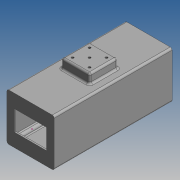
# Autodesk Inventor part: P033_Boitier_v3
Saved by Autodesk Inventor 2021.3 (Build 253353000, 353)
## iProperties
Created: 2021-11-26
Part Number: P033_Boitier_v3
Material: Générique
Document SubType Name: Modeling
Designer: gabri
Density: 1 g/cm^3
Appearance: Par défaut
Author: gabri
Autodesk Inventor part; units mm, degrees
ref_plane "YZ Plane" through (0, 0, 0) normal (1, 0, 0) x (0, 1, 0)
ref_plane "XZ Plane" through (0, 0, 0) normal (0, 1, 0) x (-1, 0, 0)
ref_plane "XY Plane" through (0, 0, 0) normal (0, 0, 1) x (1, 0, 0)
sketch "Sketch3" plane through (0, 0, 0) normal (0, 1, 0) x (-1, 0, 0)
  line L0 (-50, -50) -> (50, -50)
  line L1 (50, -50) -> (50, 50)
  line L2 (50, 50) -> (-50, 50)
  line L3 (-50, 50) -> (-50, -50)
  line L4 (-50, -50) -> (50, 50) construction
  line L5 (50, -50) -> (-50, 50) construction
  point P0 (0, 0)
  dimension "d0" = 100
  dimension "d1" = 100
  constraints: 12 end point, 2 midpoint, 2 parallel, 1 horizontal, 1 perpendicular
  measures "d0" distance between parallel lines of L3 L1
  measures "d1" distance between parallel lines of L0 L2
extrude "Extrusion1" add sketch "Sketch3" along normal blind 250
sketch "Sketch4" plane through (0, 0, 0) normal (0, -1, 0) x (1, 0, 0)
  line L0 (34, -21.5) -> (-34, -21.5)
  line L1 (-34, -21.5) -> (-34, 21.5)
  line L2 (-34, 21.5) -> (34, 21.5)
  line L3 (34, 21.5) -> (34, -21.5)
  line L4 (34, -21.5) -> (-34, 21.5) construction
  line L5 (-34, -21.5) -> (34, 21.5) construction
  point P0 (0, 0)
  dimension "d4" = 68
  dimension "d5" = 43
  constraints: 12 end point, 2 midpoint, 2 parallel, 1 horizontal, 1 perpendicular
  measures "d4" distance of L1.end L2.end
  measures "d5" distance of L0.end L1.end
extrude "Extrusion2" cut sketch "Sketch4" against normal blind 2
shell "Shell1" thickness 3 removed faces 2 at (16.6667, 250, -16.6667) at (-11.3333, 2, -7.1667)
sketch "Sketch10" plane through (0, 250, 0) normal (0, 1, 0) x (1, 0, 0)
  line L0 (-47, 47) -> (-47, -47) construction
  line L1 (-47, -47) -> (47, -47) construction
  line L2 (47, -47) -> (47, 47) construction
  line L3 (47, 47) -> (-47, 47) construction
  line L4 (-50, -50) -> (50, -50) construction
  line L5 (50, -50) -> (50, 50) construction
  line L6 (50, 50) -> (-50, 50) construction
  line L7 (-50, 50) -> (-50, -50) construction
  circle A0 centre (45, -45) radius 5
  circle A1 centre (-45, -45) radius 5
  circle A2 centre (-45, 45) radius 5
  circle A3 centre (45, 45) radius 5
  point P0 (0, 0)
  dimension "d26" = 10
  dimension "d27" = 5
  dimension "d28" = 5
  dimension "d29" = 10
  dimension "d30" = 5
  dimension "d31" = 5
  dimension "d32" = 5
  dimension "d33" = 10
  dimension "d34" = 5
  dimension "d37" = 10
  dimension "d38" = 5
  dimension "d39" = 5
  constraints: 4 centre point
  measures "d26" diameter of A0
  measures "d27" distance from line of L4 A0.centre
  measures "d28" distance from line of A0.centre L5
  measures "d29" diameter of A1
  measures "d30" distance from line of L4 A1.centre
  measures "d31" distance from line of L7 A1.centre
  measures "d32" distance from line of L7 A2.centre
  measures "d33" diameter of A2
  measures "d34" distance from line of L6 A2.centre
  measures "d37" diameter of A3
  measures "d38" distance from line of L5 A3.centre
  measures "d39" distance from line of L6 A3.centre
extrude "Extrusion5" add sketch "Sketch10" against normal up to surface (247 mm away)
sketch "Sketch11" plane through (0, 250, 0) normal (0, 1, 0) x (1, 0, 0)
  line L0 (-40.4174, 47) -> (40.4174, 47) construction
  arc A0 (40.4174, 47) -> (47, 40.4174) centre (45, 45) ccw construction
  line L1 (47, 40.4174) -> (47, -40.4174) construction
  arc A1 (47, -40.4174) -> (40.4174, -47) centre (45, -45) ccw construction
  line L2 (40.4174, -47) -> (-40.4174, -47) construction
  arc A2 (-40.4174, -47) -> (-47, -40.4174) centre (-45, -45) ccw construction
  line L3 (-47, -40.4174) -> (-47, 40.4174) construction
  arc A3 (-47, 40.4174) -> (-40.4174, 47) centre (-45, 45) ccw construction
  line L4 (50, 50) -> (-50, 50) construction
  line L5 (-50, 50) -> (-50, -50) construction
  line L6 (-50, -50) -> (50, -50) construction
  line L7 (50, -50) -> (50, 50) construction
  arc A4 (47, -40.4174) -> (40.4174, -47) centre (45, -45) ccw
  arc A5 (-40.4174, -47) -> (-47, -40.4174) centre (-45, -45) ccw
  arc A6 (-47, 40.4174) -> (-40.4174, 47) centre (-45, 45) ccw
  arc A7 (40.4174, 47) -> (47, 40.4174) centre (45, 45) ccw
  line L8 (40.4174, 47) -> (-40.4174, 47)
  line L9 (47, -40.4174) -> (47, 40.4174)
  line L10 (40.4174, -47) -> (-40.4174, -47)
  line L11 (-47, -40.4174) -> (-47, 40.4174)
  arc A8 (48, -42.3542) -> (42.3542, -48) centre (45, -45) ccw
  line L12 (42.3542, -48) -> (-42.3542, -48)
  arc A9 (-42.3542, -48) -> (-48, -42.3542) centre (-45, -45) ccw
  line L13 (-48, -42.3542) -> (-48, 42.3542)
  arc A10 (-48, 42.3542) -> (-42.3542, 48) centre (-45, 45) ccw
  line L14 (42.3542, 48) -> (-42.3542, 48)
  arc A11 (42.3542, 48) -> (48, 42.3542) centre (45, 45) ccw
  line L15 (48, -42.3542) -> (48, 42.3542)
  point P0 (0, 0)
  dimension "d45" = 1
  dimension "d46" = 4
  dimension "d47" = 1
  dimension "d48" = 4
  dimension "d49" = 1
  dimension "d50" = 4
  dimension "d51" = 1
  dimension "d54" = 4
  constraints: 17 point on circle, 16 end point, 8 centre point, 6 parallel, 4 coincident, 4 concentric, 2 collinear
  measures "d45" distance between parallel lines of L12 L10
  measures "d46" radius of A9
  measures "d47" distance between parallel lines of L13 L3
  measures "d48" radius of A10
  measures "d49" distance between parallel lines of L14 L0
  measures "d50" radius of A11
  measures "d51" distance between parallel lines of L1 L15
  measures "d54" radius of A8
extrude "Extrusion6" add sketch "Sketch11" along normal blind 2
fillet "Fillet1" radius 2 16 edges at (40.4174, 251, 47) (40.4174, 126.5, 47) (47, 251, 40.4174) (47, 126.5, 40.4174) (-40.4174, 251, 47) (-40.4174, 126.5, 47) (-47, 251, 40.4174) (-47, 126.5, 40.4174) (-47, 251, -40.4174) (-47, 126.5, -40.4174) (-40.4174, 251, -47) (-40.4174, 126.5, -47) (40.4174, 251, -47) (40.4174, 126.5, -47) (47, 251, -40.4174) (47, 126.5, -40.4174)
fillet "Fillet2" radius 2 8 edges at (42.3542, 251, -48) (48, 251, -42.3542) (48, 251, 42.3542) (42.3542, 251, 48) (-42.3542, 251, 48) (-48, 251, 42.3542) (-42.3542, 251, -48) (-48, 251, -42.3542)
fillet "Fillet3" radius 0.5 32 edges at (41.4645, 252, 41.4645) (46.4142, 252, 39.4142) (47, 252, 0) (46.4142, 252, -39.4142) (41.4645, 252, -41.4645) (39.4142, 252, -46.4142) (0, 252, -47) (-39.4142, 252, -46.4142) (-41.4645, 252, -41.4645) (-46.4142, 252, -39.4142) (-47, 252, 0) (-46.4142, 252, 39.4142) (-41.4645, 252, 41.4645) (-39.4142, 252, 46.4142) (0, 252, 47) (39.4142, 252, 46.4142) (-40.6114, 252, -47.291) (-42.1716, 252, -42.1716) (-47.291, 252, -40.6114) (-48, 252, 0) (-47.291, 252, 40.6114) (-42.1716, 252, 42.1716) (-40.6114, 252, 47.291) (0, 252, 48) (40.6114, 252, 47.291) (42.1716, 252, 42.1716) (47.291, 252, 40.6114) (48, 252, 0) (47.291, 252, -40.6114) (42.1716, 252, -42.1716) (40.6114, 252, -47.291) (0, 252, -48)
sketch "Sketch12" plane through (0, 250, 0) normal (0, 1, 0) x (1, 0, 0)
  line L0 (-39.0839, 48) -> (39.0839, 48) construction
  arc A0 (41.0559, 45.6667) -> (39.0839, 48) centre (39.0839, 46) ccw construction
  arc A1 (41.0559, 45.6667) -> (45.6667, 41.0559) centre (45, 45) ccw construction
  arc A2 (48, 39.0839) -> (45.6667, 41.0559) centre (46, 39.0839) ccw construction
  line L1 (48, 39.0839) -> (48, -39.0839) construction
  arc A3 (45.6667, -41.0559) -> (48, -39.0839) centre (46, -39.0839) ccw construction
  arc A4 (45.6667, -41.0559) -> (41.0559, -45.6667) centre (45, -45) ccw construction
  arc A5 (39.0839, -48) -> (41.0559, -45.6667) centre (39.0839, -46) ccw construction
  line L2 (39.0839, -48) -> (-39.0839, -48) construction
  arc A6 (-41.0559, -45.6667) -> (-39.0839, -48) centre (-39.0839, -46) ccw construction
  arc A7 (-41.0559, -45.6667) -> (-45.6667, -41.0559) centre (-45, -45) ccw construction
  arc A8 (-48, -39.0839) -> (-45.6667, -41.0559) centre (-46, -39.0839) ccw construction
  line L3 (-48, -39.0839) -> (-48, 39.0839) construction
  arc A9 (-45.6667, 41.0559) -> (-48, 39.0839) centre (-46, 39.0839) ccw construction
  arc A10 (-45.6667, 41.0559) -> (-41.0559, 45.6667) centre (-45, 45) ccw construction
  arc A11 (-39.0839, 48) -> (-41.0559, 45.6667) centre (-39.0839, 46) ccw construction
  line L4 (50, 50) -> (-50, 50) construction
  line L5 (-50, 50) -> (-50, -50) construction
  line L6 (-50, -50) -> (50, -50) construction
  line L7 (50, -50) -> (50, 50) construction
  point P0 (0, 0)
  constraints: 4 coincident
hole "Hole1" at (45, 250, 45) at (-45, 250, 45) at (-45, 250, -45) at (45, 250, -45) direction (0, -1, 0) diameter 4.134 depth 14.2 tip angle 118 thread size "M5x0.8" class "6H" standard "ISO Metric profile"
fillet "Fillet4" radius 4 4 edges at (-50, 125, 50) (50, 125, 50) (50, 125, -50) (-50, 125, -50)
sketch "Sketch15" plane through (-46, 0, 50) normal (0, 0, 1) x (1, 0, 0)
  line L0 (92, 250) -> (92, 0) construction
  line L1 (0, 250) -> (92, 250) construction
  line L2 (0, 0) -> (0, 250) construction
  line L3 (0, 0) -> (92, 0) construction
  line L4 (76, 95) -> (16, 95)
  line L5 (16, 95) -> (16, 155)
  line L6 (16, 155) -> (76, 155)
  line L7 (76, 155) -> (76, 95)
  line L8 (76, 95) -> (16, 155) construction
  line L9 (16, 95) -> (76, 155) construction
  line L10 (46, 302.4) -> (46, -50.4) construction
  point P0 (46, 0)
  point P1 (46, 125)
  point P2 (46, 125)
  dimension "d67" = 60
  dimension "d68" = 60
  dimension "d69" = 250
  dimension "d70" = 125
  constraints: 12 end point, 3 midpoint, 2 parallel, 1 horizontal, 1 perpendicular, 1 point on line
  measures "d67" distance between parallel lines of L7 L5
  measures "d68" distance between parallel lines of L4 L6
  measures "d69" distance between parallel lines of L3 L1
  measures "d70" distance from line of point (46, 125) L1
extrude "Extrusion7" add sketch "Sketch15" along normal blind 20
fillet "Fillet5" radius 4 12 edges at (30, 95, 60) (30, 155, 60) (-30, 155, 60) (-30, 95, 60) (-30, 125, 50) (0, 95, 50) (30, 125, 50) (0, 155, 50) (30, 125, 70) (0, 155, 70) (-30, 125, 70) (0, 95, 70)
sketch "Sketch17" plane through (-38, 3, -47) normal (0, 1, 0) x (1, 0, 0)
  point P0 (38, -47)
sketch "Sketch18" plane through (-38, 3, -47) normal (0, 1, 0) x (1, 0, 0)
  line L0 (1, -22.5) -> (1, -71.5) construction
  line L1 (75, -22.5) -> (1, -22.5) construction
  line L2 (75, -71.5) -> (75, -22.5) construction
  line L3 (1, -71.5) -> (75, -71.5) construction
  arc A0 (85, -9) -> (83, -7) centre (83, -9) ccw construction
  arc A1 (78, -2) -> (83, -7) centre (83, -2) ccw construction
  arc A2 (78, -2) -> (76, 0) centre (76, -2) ccw construction
  line L4 (76, 0) -> (0, 0) construction
  arc A3 (0, 0) -> (-2, -2) centre (0, -2) ccw construction
  arc A4 (-7, -7) -> (-2, -2) centre (-7, -2) ccw construction
  arc A5 (-7, -7) -> (-9, -9) centre (-7, -9) ccw construction
  line L5 (-9, -9) -> (-9, -85) construction
  arc A6 (-9, -85) -> (-7, -87) centre (-7, -85) ccw construction
  arc A7 (-2, -92) -> (-7, -87) centre (-7, -92) ccw construction
  arc A8 (-2, -92) -> (0, -94) centre (0, -92) ccw construction
  line L6 (0, -94) -> (76, -94) construction
  arc A9 (76, -94) -> (78, -92) centre (76, -92) ccw construction
  arc A10 (83, -87) -> (78, -92) centre (83, -92) ccw construction
  arc A11 (83, -87) -> (85, -85) centre (83, -85) ccw construction
  line L7 (85, -85) -> (85, -9) construction
  arc A12 (-2, -92) -> (-7, -87) centre (-7, -92) ccw
  arc A13 (-2, -92) -> (0, -94) centre (0, -92) ccw
  arc A14 (83, -87) -> (78, -92) centre (83, -92) ccw
  arc A15 (76, -94) -> (78, -92) centre (76, -92) ccw
  line L8 (76, -94) -> (0, -94)
  line L9 (-7, -87) -> (83, -87)
  point P0 (38, -47)
  constraints: 11 point on circle, 4 centre point, 4 end point, 3 concentric, 2 tangent, 1 collinear, 1 horizontal
extrude "Extrusion8" add sketch "Sketch18" along normal up to surface (247 mm away)
sketch "Sketch19" plane through (-46, 0, 70) normal (0, 0, 1) x (1, 0, 0)
  line L0 (72, 151) -> (72, 99) construction
  line L1 (20, 151) -> (72, 151) construction
  line L2 (20, 99) -> (20, 151) construction
  line L3 (72, 99) -> (20, 99) construction
  line L4 (46, 302.4) -> (46, -50.4) construction
  line L5 (-24, 0) -> (116, 0) construction
  point P0 (46, 0)
  point P1 (28, 143)
  point P2 (46, 125)
  point P3 (64, 143)
  point P4 (28, 107)
  point P5 (64, 107)
  dimension "d77" = 52
  dimension "d78" = 52
  dimension "d79" = 8
  dimension "d80" = 8
  dimension "d84" = 36
  dimension "d87" = 36
  dimension "d90" = 125
  constraints: 1 horizontal, 1 point on line, 1 vertical, 3 other
  measures "d77" distance between parallel lines of L0 L2
  measures "d78" distance between parallel lines of L3 L1
  measures "d79" distance from line of L1 point (28, 143)
  measures "d80" distance from line of L2 point (28, 143)
  measures "d84" distance of point (28, 143) point (64, 143)
  measures "d87" distance of point (28, 143) point (28, 107)
  measures "d90" distance from line of L5 point (46, 125)
hole "Hole2" at (-18, 143, 70) at (18, 143, 70) at (18, 107, 70) at (-18, 107, 70) at (0, 125, 70) direction (0, 0, -1) diameter 4.917 depth 17.1 tip angle 118 thread size "M6x1" class "6H" standard "ISO Metric profile"
sketch "Sketch20" plane through (-37, 2, 24.5) normal (0, 1, 0) x (1, 0, 0)
  line L0 (3, 46) -> (3, 3) construction
  line L1 (71, 46) -> (3, 46) construction
  line L2 (71, 3) -> (71, 46) construction
  line L3 (3, 3) -> (71, 3) construction
  line L4 (0, 0) -> (74, 0) construction
  line L5 (74, 0) -> (74, 49) construction
  line L6 (74, 49) -> (0, 49) construction
  line L7 (0, 49) -> (0, 0) construction
  line L8 (74, 0) -> (0, 0)
  line L9 (0, 0) -> (0, 49)
  line L10 (0, 49) -> (74, 49)
  line L11 (74, 49) -> (74, 0)
  line L12 (74, 0) -> (0, 49) construction
  line L13 (0, 0) -> (74, 49) construction
  line L14 (71, 3) -> (3, 3)
  line L15 (3, 3) -> (3, 46)
  line L16 (3, 46) -> (71, 46)
  line L17 (71, 46) -> (71, 3)
  line L18 (71, 3) -> (3, 46) construction
  line L19 (3, 3) -> (71, 46) construction
  point P0 (37, 24.5)
  constraints: 24 end point, 4 midpoint, 4 parallel, 2 horizontal, 2 perpendicular
extrude "Extrusion9" add sketch "Sketch20" along normal up to surface (1 mm away)
equation "\"d27\" = 0.5 * d26"
equation "\"d28\" = 0.5 * d26"
equation "\"d30\" = 0.5 * d29"
equation "\"d31\" = 0.5 * d29"
equation "\"d32\" = 0.5 * d33"
equation "\"d34\" = 0.5 * d33"
equation "\"d38\" = 0.5 * d37"
equation "\"d39\" = 0.5 * d37"
equation "\"d70\" = 0.5 * d69"
body "Solid1"
